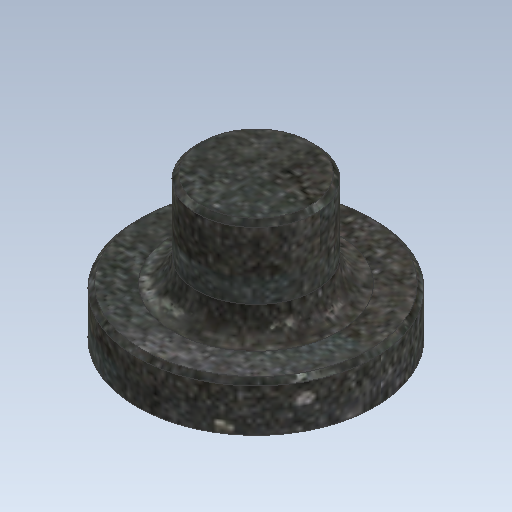
# Autodesk Inventor part: Projekt elementy
Saved by Autodesk Inventor 2021 (Build 250183000, 183)
## iProperties
Created: 2020-04-11
Part Number: Projekt elementy
Material: Stal
Document SubType Name: Modeling
Designer: dyrag
Mass: 220.666 g
Surface Area: 74.1888 cm^2
Volume: 28.1103 cm^3
Density: 7.85 g/cm^3
Appearance: Płyta
Author: dyrag
Autodesk Inventor part; units mm, degrees
ref_plane "YZ Plane" through (0, 0, 0) normal (1, 0, 0) x (0, 1, 0)
ref_plane "XZ Plane" through (0, 0, 0) normal (0, 1, 0) x (-1, 0, 0)
ref_plane "XY Plane" through (0, 0, 0) normal (0, 0, 1) x (1, 0, 0)
sketch "Szkic1" plane through (0, 0, 0) normal (0, 0, 1) x (1, 0, 0)
  line L0 (0, 0) -> (0, 30)
  line L1 (0, 30) -> (-12.5, 30)
  line L2 (-12.5, 30) -> (-12.5, 10)
  line L3 (-12.5, 10) -> (-25, 10)
  line L4 (-25, 10) -> (-25, 0)
  line L5 (-25, 0) -> (0, 0)
  constraints: 12 end point, 3 perpendicular, 1 horizontal, 1 vertical
revolve "Obrót1" add sketch "Szkic1" angle 360 about axis through (0, 0, 0) along (0, 1, 0)
fillet "Zaokrąglenie1" radius 5 1 edges at (12.5, 10, 0)
chamfer "Faza1" distance 1 angle 45 2 edges at (12.5, 30, 0) (25, 10, 0)
sketch "Szkic2" plane through (0, 0, 0) normal (0, -1, 0) x (1, 0, 0)
  point P0 (0, 0)
hole "Otwór1" at (0, 0, 0) direction (0, 1, 0) diameter 10.106 depth 20 tip angle 118 thread size "M12x1.75" class "6H" standard "ISO Metric profile"
